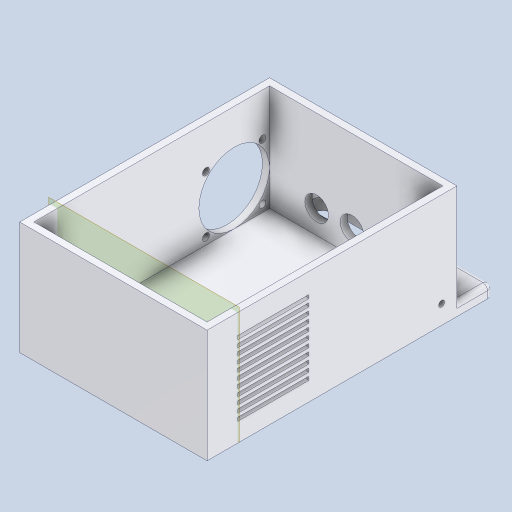
# Autodesk Inventor part: Controller Enclosure
Saved by Autodesk Inventor 2024 (Build 280153000, 153)
## iProperties
Created: 2025-03-05
Part Number: Controller Enclosure
Material: Generic
Document SubType Name: Modeling
Designer: Kemper Room 121
Density: 1 g/cm^3
Appearance: PTFE
Author: Kemper Room 121
Autodesk Inventor part; units mm, degrees
ref_plane "YZ Plane" through (0, 0, 0) normal (1, 0, 0) x (0, 1, 0)
ref_plane "XZ Plane" through (0, 0, 0) normal (0, 1, 0) x (-1, 0, 0)
ref_plane "XY Plane" through (0, 0, 0) normal (0, 0, 1) x (1, 0, 0)
sketch "Sketch1" plane through (0, 0, 0) normal (0, 1, 0) x (-1, 0, 0)
  line L0 (0, 0) -> (-51.5, 0)
  line L1 (-51.5, 0) -> (-51.5, -100)
  line L2 (-51.5, -100) -> (0, -100)
  line L3 (0, -100) -> (0, 0)
  circle A0 centre (-4, -4) radius 1.625
  circle A1 centre (-47.5, -11.5) radius 1.625
  dimension "d0" = 51.5
  dimension "d1" = 100
  dimension "d2" = 3.25
  dimension "d3" = 3.25
  dimension "d4" = 4
  dimension "d5" = 4
  dimension "d6" = 4
  dimension "d7" = 11.5
  constraints: 8 end point, 2 centre point, 2 parallel, 1 horizontal, 1 perpendicular
  measures "d0" distance of L0.start L0.end
  measures "d1" distance of L2.end L0.start
  measures "d2" diameter of A1
  measures "d3" diameter of A0
  measures "d4" distance from line of L0 A0.centre
  measures "d5" distance from line of L3 A0.centre
  measures "d6" distance from line of L1 A1.centre
  measures "d7" distance from line of L0 A1.centre
extrude "Extrusion1" add sketch "Sketch1" against normal blind 1
sketch "Sketch2" plane through (0, 0, 0) normal (0, 1, 0) x (1, 0, 0)
  line L0 (21.5, 4) -> (73.5, 4)
  line L1 (73.5, 4) -> (73.5, 93)
  line L2 (73.5, 93) -> (21.5, 93)
  line L3 (21.5, 93) -> (21.5, 4)
  circle A0 centre (47.5, 11.5) radius 1.625
  circle A1 centre (29.75, 12.25) radius 1.125
  line L4 (51.5, 0) -> (51.5, 100) projected
  line L5 (51.5, 100) -> (0, 100) projected
  line L6 (0, 100) -> (0, 0) projected
  line L7 (0, 0) -> (51.5, 0) projected
  circle A2 centre (4, 4) radius 1.625 projected
  circle A3 centre (47.5, 11.5) radius 1.625 projected
  point P0 (47.5, 4)
  dimension "d10" = 3.25
  dimension "d11" = 52
  dimension "d12" = 89
  dimension "d13" = 2.25
  dimension "d14" = 8.25
  dimension "d15" = 8.25
  dimension "d16" = 0
  dimension "d17" = 7.5
  dimension "d18" = 0
  dimension "d19" = 0
  constraints: 8 end point, 2 centre point, 2 parallel, 1 horizontal, 1 midpoint, 1 perpendicular
  measures "d10" diameter of A0
  measures "d11" distance of L0.start L0.end
  measures "d12" distance of L2.end L0.start
  measures "d13" diameter of A1
  measures "d14" distance from line of L3 A1.centre
  measures "d15" distance from line of L0 A1.centre
  measures "d16" horizontal distance of point (47.5, 4) A0.centre
  measures "d17" distance from line of L0 A0.centre
  measures "d18" distance of A3.centre A0.centre
  measures "d19" distance of A3.centre A0.centre
extrude "Extrusion2" add sketch "Sketch2" against normal blind 1 contours L3 L2 L4 L0 | L4 L2 L1 L0
sketch "Sketch3" plane through (0, 0, 0) normal (0, 1, 0) x (1, 0, 0)
  line L0 (51.5, 4) -> (73.5, 4) projected
  line L1 (73.5, 4) -> (73.5, 93) projected
  line L2 (73.5, 93) -> (51.5, 93) projected
  line L3 (51.5, 100) -> (0, 100) projected
  line L4 (0, 100) -> (0, 0) projected
  line L5 (0, 0) -> (51.5, 0) projected
  line L6 (51.5, 0) -> (51.5, 4) projected
  circle A0 centre (4, 4) radius 1.625 projected
  circle A1 centre (47.5, 11.5) radius 1.625 projected
  line L7 (-3, -3) -> (76.5, -3)
  line L8 (76.5, -3) -> (76.5, 103)
  line L9 (76.5, 103) -> (-3, 103)
  line L10 (-3, 103) -> (-3, -3)
  line L11 (51.5, 93) -> (51.5, 100) projected
  dimension "d22" = 3
  dimension "d23" = 3
  dimension "d24" = 3
  dimension "d48" = 3
  constraints: 8 end point, 2 parallel, 1 horizontal, 1 perpendicular
  measures "d22" distance between parallel lines of L4 L10
  measures "d23" distance between parallel lines of L5 L7
  measures "d24" distance between parallel lines of L1 L8
  measures "d48" distance between parallel lines of L3 L9
extrude "Extrusion3" add sketch "Sketch3" along normal blind 3 contours L6 L5 L4 L3 L11 L2 L1 L0 | A0 | A1 | L10 L9 L8 L7
sketch "Sketch4" plane through (0, 3, 0) normal (0, 1, 0) x (1, 0, 0)
  line L0 (76.5, -3) -> (76.5, 103) projected
  line L1 (76.5, 103) -> (-3, 103) projected
  line L2 (-3, 103) -> (-3, -3) projected
  line L3 (-3, -3) -> (76.5, -3) projected
  line L4 (-3, 103) -> (76.5, 103)
  line L5 (76.5, 103) -> (76.5, -3)
  line L6 (76.5, -3) -> (-3, -3)
  line L7 (-3, -3) -> (-3, 103)
  line L8 (0, 100) -> (73.5, 100)
  line L9 (73.5, 100) -> (73.5, 0)
  line L10 (73.5, 0) -> (0, 0)
  line L11 (0, 0) -> (0, 100)
  point P0 (0, 0)
  dimension "d28" = 3
  dimension "d29" = 3
  dimension "d30" = 3
  dimension "d31" = 3
  constraints: 16 end point, 4 parallel, 2 horizontal, 2 perpendicular
  measures "d28" distance between parallel lines of L0 L9
  measures "d29" distance between parallel lines of L2 L11
  measures "d30" distance between parallel lines of L3 L10
  measures "d31" distance between parallel lines of L1 L8
extrude "Extrusion4" add sketch "Sketch4" along normal blind 45
sketch "Sketch5" plane through (0, 3, 0) normal (0, 1, 0) x (1, 0, 0)
  circle A0 centre (47.5, 11.5) radius 4
  line L0 (73.5, 0) -> (0, 0) projected
  line L1 (0, 0) -> (0, 100) projected
  circle A1 centre (47.5, 85.5) radius 4
  line L2 (0, 100) -> (73.5, 100) projected
  circle A2 centre (4, 4) radius 1.625 projected
  circle A3 centre (4, 4) radius 4
  dimension "d34" = 8
  dimension "d36" = 11.5
  dimension "d37" = 47.5
  dimension "d39" = 8
  dimension "d42" = 74
  dimension "d45" = 8
  constraints: 3 centre point, 1 coincident
  measures "d34" diameter of A0
  measures "d36" distance from line of L0 A0.centre
  measures "d37" distance from line of L1 A0.centre
  measures "d39" diameter of A1
  measures "d42" distance of A0.centre A1.centre
  measures "d45" diameter of A3
extrude "Extrusion5" add sketch "Sketch5" along normal blind 5 contours A0 | A3 | A1 | A2
sketch "Sketch6" plane through (47.5, 8, -85.5) normal (0, 1, 0) x (1, 0, 0)
  circle A0 centre (0, 0) radius 4 projected
  circle A1 centre (0, 0) radius 3
  point P0 (-47.5, -85.5)
  constraints: 1 centre point, 1 coincident
extrude "Extrusion6" add sketch "Sketch6" along normal blind 1.5 contours A0 | A1
sketch "Sketch7" plane through (0, 3, 0) normal (1, 0, 0) x (0, 0, -1)
  line L0 (100, 0) -> (4, 0) projected
  line L1 (100, 0) -> (100, 45) projected
  line L2 (0, 45) -> (100, 45) projected
  line L3 (0, 0) -> (0, 45) projected
  line L4 (100, 0) -> (70, 0)
  line L5 (70, 0) -> (70, 30)
  line L6 (70, 30) -> (100, 30)
  line L7 (100, 30) -> (100, 0)
  circle A0 centre (85, 15) radius 15
  circle A1 centre (73, 27) radius 1.5
  circle A2 centre (97, 27) radius 1.5
  circle A3 centre (73, 3) radius 1.5
  circle A4 centre (97, 3) radius 1.5
  line L8 (4, 0) -> (0, 0) projected
  line L9 (4, 0) -> (4, 5) projected
  point P0 (0, -3)
  point P1 (70, 15)
  point P2 (85, 30)
  point P3 (70, 15)
  point P4 (70, 0)
  point P5 (85, 0)
  point P6 (75.081, 3.7477)
  point P7 (74.196, 4.5945)
  dimension "d49" = 30
  dimension "d50" = 30
  dimension "d51" = 0
  dimension "d52" = 0
  dimension "d53" = 30
  dimension "d54" = 24
  dimension "d55" = 3
  dimension "d56" = 12
  dimension "d57" = 3
  dimension "d58" = 24
  dimension "d59" = 24
  dimension "d60" = 24
  dimension "d61" = 3
  dimension "d62" = 3
  dimension "d65" = 0
  dimension "d90" = 12
  dimension "d91" = 0
  constraints: 8 end point, 5 centre point, 2 midpoint, 2 parallel, 1 horizontal, 1 perpendicular
  measures "d49" distance of L4.end L5.end
  measures "d50" distance of L5.end L6.end
  measures "d51" vertical distance of point (70, 15) A0.centre
  measures "d52" horizontal distance of point (85, 30) A0.centre
  measures "d53" diameter of A0
  measures "d54" distance of A1.centre A2.centre
  measures "d55" diameter of A1
  measures "d56" horizontal distance of A0.centre A1.centre
  measures "d57" diameter of A2
  measures "d58" distance of A1.centre A3.centre
  measures "d59" distance of A3.centre A4.centre
  measures "d60" distance of A4.centre A2.centre
  measures "d61" diameter of A4
  measures "d62" diameter of A3
  measures "d65" horizontal distance of A1.centre A3.centre
  measures "d90" horizontal distance of A0.centre A1.centre
  measures "d91" vertical distance of A2.centre A1.centre
extrude "Extrusion7" cut sketch "Sketch7" against normal blind 30 contours A0 | A1 | A2 | A3 | A4
sketch "Sketch8" plane through (0, 48, 0) normal (0, 1, 0) x (1, 0, 0)
  line L0 (0, 100) -> (73.5, 100) projected
  line L1 (73.5, 100) -> (73.5, 0) projected
  line L2 (73.5, 0) -> (0, 0) projected
  line L3 (0, 0) -> (0, 100) projected
  line L4 (-3, 103) -> (-3, -3) projected
  line L5 (-3, -3) -> (76.5, -3) projected
  line L6 (76.5, -3) -> (76.5, 103) projected
  line L7 (76.5, 103) -> (-3, 103) projected
  line L8 (76.5, -3) -> (76.5, 103) projected
  line L9 (-3, -3) -> (76.5, -3)
  line L10 (76.5, -3) -> (76.5, 103)
  line L11 (76.5, 103) -> (-3, 103)
  line L12 (-3, 103) -> (-3, -3)
  line L13 (73.5, 0) -> (73.5, 100) projected
  line L14 (0, 0) -> (73.5, 0)
  line L15 (73.5, 0) -> (73.5, 100)
  line L16 (73.5, 100) -> (0, 100)
  line L17 (0, 100) -> (0, 0)
  point P0 (0, 0)
  constraints: 16 end point, 4 parallel, 2 horizontal, 2 perpendicular
extrude "Extrusion8" [suppressed]
sketch "Sketch9" plane through (0, 51, 0) normal (0, 1, 0) x (1, 0, 0)
  line L0 (-3, -3) -> (76.5, -3) projected
  line L1 (76.5, -3) -> (76.5, 103) projected
  line L2 (76.5, 103) -> (-3, 103) projected
  line L3 (-3, 103) -> (-3, -3) projected
  line L4 (0, 100) -> (10, 100)
  line L5 (10, 100) -> (10, 90)
  line L6 (10, 90) -> (0, 90)
  line L7 (0, 90) -> (0, 100)
  line L8 (73.5, 100) -> (63.5, 100)
  line L9 (63.5, 100) -> (63.5, 90)
  line L10 (63.5, 90) -> (73.5, 90)
  line L11 (73.5, 90) -> (73.5, 100)
  line L12 (0, 0) -> (10, 0)
  line L13 (10, 0) -> (10, 10)
  line L14 (10, 10) -> (0, 10)
  line L15 (0, 10) -> (0, 0)
  line L16 (73.5, 0) -> (63.5, 0)
  line L17 (63.5, 0) -> (63.5, 10)
  line L18 (63.5, 10) -> (73.5, 10)
  line L19 (73.5, 10) -> (73.5, 0)
  point P0 (0, 0)
  dimension "d68" = 10
  dimension "d69" = 10
  dimension "d70" = 10
  dimension "d71" = 10
  dimension "d72" = 10
  dimension "d73" = 10
  dimension "d74" = 10
  dimension "d75" = 10
  constraints: 32 end point, 8 parallel, 4 horizontal, 4 perpendicular
  measures "d68" distance of L5.end L6.end
  measures "d69" distance of L4.end L5.end
  measures "d70" distance of L8.end L9.end
  measures "d71" distance of L9.end L10.end
  measures "d72" distance of L13.end L14.end
  measures "d73" distance of L12.end L13.end
  measures "d74" distance of L16.end L17.end
  measures "d75" distance of L17.end L18.end
extrude "Extrusion10" [suppressed]
sketch "Sketch11" plane through (0, 3, 0) normal (0, 1, 0) x (1, 0, 0)
  circle A0 centre (47.5, 85.5) radius 4 projected
  circle A1 centre (47.5, 11.5) radius 4 projected
  arc A2 (4, 0) -> (0, 4) centre (4, 4) ccw projected
  line L0 (0, 100) -> (0, 85) projected
  line L1 (0, 85) -> (0, 4) projected
  line L2 (0, 0) -> (4, 0) projected
  line L3 (73.5, 0) -> (73.5, 100) projected
  line L4 (73.5, 100) -> (0, 100) projected
  line L5 (73.5, 100) -> (63.5, 100)
  line L6 (63.5, 100) -> (63.5, 86)
  line L7 (63.5, 86) -> (73.5, 86)
  line L8 (73.5, 86) -> (73.5, 100)
  line L9 (53.5, 100) -> (63.5, 100)
  line L10 (63.5, 100) -> (63.5, 86)
  line L11 (63.5, 86) -> (73.5, 86)
  line L12 (73.5, 86) -> (73.5, 80)
  line L13 (4, 0) -> (73.5, 0) projected
  arc A3 (0, 4) -> (4, 0) centre (4, 4) ccw projected
  line L14 (0, 4) -> (0, 0) projected
  point P0 (0, 0)
  dimension "d95" = 10
  dimension "d100" = 14
  constraints: 16 end point, 2 horizontal, 2 parallel, 2 perpendicular, 2 point on line
  measures "d95" distance of L6.end L7.end
  measures "d100" distance of L5.end L6.end
extrude "Extrusion11" add sketch "Sketch11" along normal blind 10 contours L7 L6 L4 L3
sketch "Sketch12" plane through (63.5, 3, -100) normal (-1, 0, 0) x (0, 0, 1)
  line L0 (14, 0) -> (0, 0) projected
  line L1 (14, 0) -> (14, 10) projected
  line L2 (0, 10) -> (14, 10) projected
  line L3 (0, 0) -> (0, 10) projected
  circle A0 centre (3.5, 5) radius 1.25
  line L4 (0, 10) -> (14, 10) projected
  point P0 (100, -3)
  point P1 (7, 10)
  point P2 (7, 10)
  dimension "d101" = 2.5
  dimension "d104" = 5
  dimension "d112" = 3.5
  constraints: 2 midpoint, 1 centre point
  measures "d101" diameter of A0
  measures "d104" distance from line of L0 A0.centre
  measures "d112" distance from line of L3 A0.centre
extrude "Extrusion12" cut sketch "Sketch12" against normal through all contours A0
sketch "Sketch13" plane through (0, 13, 0) normal (0, 1, 0) x (1, 0, 0)
  line L0 (73.5, 100) -> (73.5, 86) projected
  line L1 (63.5, 100) -> (73.5, 100) projected
  line L2 (63.5, 100) -> (63.5, 86) projected
  line L3 (63.5, 86) -> (73.5, 86) projected
  line L4 (70, 100) -> (73.5, 100)
  line L5 (73.5, 100) -> (73.5, 92.5)
  line L6 (73.5, 92.5) -> (70, 92.5)
  line L7 (70, 92.5) -> (70, 100)
  point P0 (0, 0)
  dimension "d108" = 3.5
  dimension "d113" = 7.5
  constraints: 8 end point, 2 parallel, 2 point on line, 1 horizontal, 1 perpendicular
  measures "d108" distance of L5.end L6.end
  measures "d113" distance of L6.end L4.start
extrude "Extrusion13" cut sketch "Sketch13" against normal blind 10 contours L0 L6 L7 L1
sketch "Sketch14" plane through (76.5, 0, -103) normal (0, 0, -1) x (-1, 0, 0)
  line L0 (13, 3) -> (13, 13) projected
  line L1 (13, 13) -> (6.5, 13) projected
  line L2 (3, 3) -> (3, 48) projected
  line L3 (76.5, 18) -> (76.5, 48) projected
  line L4 (76.5, 3) -> (76.5, 18) projected
  line L5 (13, 3) -> (76.5, 3) projected
  circle A0 centre (26.5, 13) radius 5
  circle A1 centre (41.5, 13) radius 5
  circle A2 centre (56.5, 13) radius 5
  line L6 (76.5, 48) -> (3, 48) projected
  line L7 (6.5, 13) -> (6.5, 3) projected
  line L8 (6.5, 3) -> (3, 3) projected
  point P0 (76.5, 0)
  dimension "d114" = 10
  dimension "d124" = 15
  dimension "d129" = 10
  dimension "d131" = 20
  constraints: 3 centre point
  measures "d114" diameter of A0
  measures "d124" distance of A0.centre A1.centre
  measures "d129" distance from line of L5 A0.centre
  measures "d131" distance from line of L4 A2.centre
extrude "Extrusion14" cut sketch "Sketch14" against normal blind 10 contours A0 | A1 | A2
sketch "Sketch15" plane through (47.5, 9.5, -85.5) normal (0, 1, 0) x (1, 0, 0)
  circle A0 centre (0, 0) radius 4 projected
  circle A1 centre (-43.5, -81.5) radius 1.625 projected
  circle A2 centre (0, -74) radius 4 projected
  circle A3 centre (0, 0) radius 2.1
  circle A4 centre (-43.5, -81.5) radius 2.1
  circle A5 centre (0, -74) radius 1.625 projected
  circle A6 centre (0, -74) radius 2.1
  point P0 (-47.5, -85.5)
  dimension "d134" = 4.2
  dimension "d135" = 4.2
  dimension "d136" = 4.2
  constraints: 3 centre point, 3 coincident
  measures "d134" diameter of A3
  measures "d135" diameter of A4
  measures "d136" diameter of A6
extrude "Extrusion15" cut sketch "Sketch15" against normal blind 5 contours A1 | A3 | A4 | A5 | A6
sketch "Sketch16" plane through (76.5, 0, -103) normal (0, 0, -1) x (-1, 0, 0)
  line L0 (0, 0) -> (79.5, 0) projected
  line L1 (79.5, 0) -> (79.5, 48) projected
  line L2 (0, 0) -> (0, 48) projected
  line L3 (0, 0) -> (79.5, 0)
  line L4 (79.5, 0) -> (79.5, 5)
  line L5 (79.5, 5) -> (0, 5)
  line L6 (0, 5) -> (0, 0)
  line L7 (0, 48) -> (79.5, 48) projected
  point P0 (76.5, 0)
  point P1 (0, 5)
  dimension "d139" = 5
  constraints: 8 end point, 2 parallel, 1 horizontal, 1 perpendicular, 1 point on line
  measures "d139" distance between parallel lines of L0 L5
extrude "Extrusion16" add sketch "Sketch16" along normal blind 15 contours L2 L5 L1 L0
sketch "Sketch17" plane through (-3, 5, -103) normal (0, 1, 0) x (1, 0, 0)
  line L0 (79.5, 0) -> (0, 0) projected
  line L1 (79.5, 0) -> (79.5, 15) projected
  line L2 (0, 15) -> (79.5, 15) projected
  line L3 (0, 0) -> (0, 15) projected
  circle A0 centre (15, 7.5) radius 4.175
  circle A1 centre (64.5, 7.5) radius 4.175
  line L4 (15, 3.325) -> (64.5, 3.325)
  line L5 (64.5, 3.325) -> (64.5, 11.675)
  line L6 (64.5, 11.675) -> (15, 11.675)
  line L7 (15, 11.675) -> (15, 3.325)
  point P0 (3, -103)
  point P1 (15, 7.5)
  point P2 (64.5, 3.325)
  point P3 (15, 11.675)
  dimension "d142" = 8.35
  dimension "d143" = 8.35
  dimension "d144" = 15
  dimension "d145" = 15
  dimension "d146" = 0
  constraints: 8 end point, 2 midpoint, 2 parallel, 1 horizontal, 1 perpendicular, 6 other
  measures "d144" distance from line of L3 point (15, 7.5)
  measures "d145" distance from line of L1 point (64.5, 7.5)
  measures "d146" distance of point (64.5, 7.5) point (64.5, 7.5)
extrude "Extrusion17" cut sketch "Sketch17" against normal blind 15 contours A0 L7 | A0 L6 A1 L4 | L7 A0 | L5 A1 | A1 L5
fillet "Fillet1" radius 2 5 edges at (76.5, 2.5, -118) (-3, 2.5, -118) (76.5, 5, -110.5) (36.75, 5, -118) (-3, 5, -110.5)
sketch "Sketch18" plane through (0, 0, 0) normal (0, -1, 0) x (1, 0, 0)
  line L0 (-42.8807, 22.4095) -> (141.815, 22.4095)
  line L1 (141.815, 22.4095) -> (141.815, -149.6316)
  line L2 (141.815, -149.6316) -> (-42.8807, -149.6316)
  line L3 (-42.8807, -149.6316) -> (-42.8807, 22.4095)
  point P0 (0, 0)
  constraints: 8 end point, 2 parallel, 1 horizontal, 1 perpendicular
extrude "Extrusion18" cut sketch "Sketch18" along normal blind 10
ref_plane "Work Plane2" through (73.5, 48, -10) normal (0, 0, -1) x (-1, 0, 0)
sketch "Sketch19" plane through (73.5, 48, -10) normal (0, 0, -1) x (-1, 0, 0)
  line L0 (73.5, -45) -> (69.5, -45) projected
  line L1 (73.5, -45) -> (73.5, 0) projected
  line L2 (0, 0) -> (73.5, 0) projected
  line L3 (0, -45) -> (0, 0) projected
  line L4 (69.5, -45) -> (0, -45) projected
  line L5 (69.5, -45) -> (69.5, -40) projected
  line L6 (-1, -43) -> (74.5, -43) projected
  arc A0 (76.5, -45) -> (74.5, -43) centre (74.5, -45) ccw projected
  line L7 (76.5, -45) -> (76.5, 0) projected
  line L8 (-3, 0) -> (76.5, 0) projected
  line L9 (-3, -45) -> (-3, 0) projected
  arc A1 (-1, -43) -> (-3, -45) centre (-1, -45) ccw projected
  circle A2 centre (53.5, -35) radius 5 projected
  circle A3 centre (38.5, -35) radius 5 projected
  circle A4 centre (23.5, -35) radius 5 projected
  line L10 (0, -45) -> (-3, -45)
  line L11 (-3, -45) -> (-3, -40)
  line L12 (-3, -40) -> (0, -40)
  line L13 (0, -40) -> (0, -45)
  line L14 (-3, -40) -> (0, -38.2679)
  line L15 (-3, -38.5) -> (0, -36.7679)
  line L16 (-3, -37) -> (0, -35.2679)
  line L17 (-3, -35.5) -> (0, -33.7679)
  line L18 (-3, -34) -> (0, -32.2679)
  line L19 (-3, -32.5) -> (0, -30.7679)
  line L20 (-3, -31) -> (0, -29.2679)
  line L21 (-3, -29.5) -> (0, -27.7679)
  line L22 (-3, -28) -> (0, -26.2679)
  line L23 (-3, -26.5) -> (0, -24.7679)
  line L24 (-3, -25) -> (0, -23.2679)
  line L25 (-3, -23.5) -> (0, -21.7679)
  line L26 (-3, -22) -> (0, -20.2679)
  line L27 (-3, -20.5) -> (0, -18.7679)
  line L28 (-3, -19) -> (0, -17.2679)
  line L29 (-3, -17.5) -> (0, -15.7679)
  line L30 (-3, -16) -> (0, -14.2679)
  line L31 (-3, -14.5) -> (0, -12.7679)
  line L32 (-3, -13) -> (0, -11.2679)
  line L33 (-3, -11.5) -> (0, -9.7679)
  line L34 (-3, -10) -> (0, -8.2679)
  line L35 (-3, -8.5) -> (0, -6.7679)
  line L36 (-3, -7) -> (0, -5.2679)
  line L37 (-3, -5.5) -> (0, -3.7679)
  line L38 (-3, -4) -> (0, -2.2679)
  line L39 (-3, -2.5) -> (0, -0.7679)
  line L40 (-3, -40) -> (0, -40)
  line L41 (0, -40) -> (0, 0)
  line L42 (0, 0) -> (-3, 0)
  line L43 (-3, 0) -> (-3, -40)
  point P0 (73.5, -48)
  point P1 (-1.5, -45)
  point P2 (-1.5, -40)
  point P3 (0, -6.7679)
  point P4 (-3, -8.5)
  point P5 (-3, -10)
  point P6 (0, -8.2679)
  point P7 (0, -9.7679)
  point P8 (-3, -11.5)
  point P9 (-3, -13)
  point P10 (0, -11.2679)
  point P11 (0, -12.7679)
  point P12 (-3, -14.5)
  point P13 (-3, -16)
  point P14 (0, -14.2679)
  point P15 (0, -15.7679)
  point P16 (-3, -17.5)
  point P17 (-3, -19)
  point P18 (0, -17.2679)
  point P19 (0, -18.7679)
  point P20 (-3, -20.5)
  point P21 (-3, -22)
  point P22 (0, -20.2679)
  point P23 (0, -21.7679)
  point P24 (-3, -23.5)
  point P25 (-3, -25)
  point P26 (0, -23.2679)
  point P27 (0, -24.7679)
  point P28 (-3, -26.5)
  point P29 (-3, -28)
  point P30 (0, -26.2679)
  point P31 (0, -27.7679)
  point P32 (-3, -29.5)
  point P33 (-3, -31)
  point P34 (0, -29.2679)
  point P35 (0, -30.7679)
  point P36 (-3, -32.5)
  point P37 (-3, -34)
  point P38 (0, -32.2679)
  point P39 (0, -33.7679)
  point P40 (-3, -35.5)
  point P41 (-3, -37)
  point P42 (0, -35.2679)
  dimension "d153" = 5
  dimension "d154" = 30
  dimension "d155" = 1.5
  dimension "d156" = 1.5
  dimension "d159" = 3
  constraints: 68 end point, 48 vertical alignment, 29 parallel, 2 horizontal, 2 midpoint, 2 perpendicular, 6 other
  measures "d153" distance of point (-1.5, -45) point (-1.5, -40)
  measures "d154" angle of L12 L14
  measures "d155" distance of L11.end L15.start
  measures "d156" distance of L15.end L14.end
  measures "d159" distance of L11.end L16.start
extrude "Extrusion19" cut sketch "Sketch19" along normal blind 30 contours L9 L15 L3 L14 | L9 L17 L3 L16 | L9 L19 L3 L18 | L3 L34 L9 L35 | L9 L21 L3 L20 | L3 L32 L9 L33 | L9 L23 L3 L22 | L3 L30 L9 L31 | L9 L25 L3 L24 | L3 L28 L9 L29 | L9 L27 L3 L26
equation "\"d2\" = d3"
equation "\"d6\" = d5"
equation "\"d34\" = d45"
equation "\"d39\" = d45"
equation "\"d56\" = 0.5 * d54"
equation "\"d57\" = d55"
equation "\"d58\" = d54"
equation "\"d59\" = d54"
equation "\"d60\" = d54"
equation "\"d61\" = d55"
equation "\"d62\" = d55"
equation "\"d90\" = 0.5 * d58"
equation "\"d70\" = d69"
equation "\"d71\" = d68"
equation "\"d72\" = d68"
equation "\"d73\" = d69"
equation "\"d74\" = d70"
equation "\"d75\" = d71"
equation "\"d143\" = d142"
body "Solid1"
